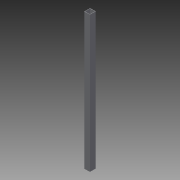
# Autodesk Inventor part: Edge Mount Interference
Saved by Autodesk Inventor 2013 (Build 170138000, 138)
## iProperties
Created: 2013-01-23
Part Number: Edge Mount Interference
Material: Generic
Document SubType Name: Modeling
Designer: actoennies
Density: 1 g/cm^3
Author: actoennies
Autodesk Inventor part; units mm, degrees
ref_plane "YZ Plane" through (0, 0, 0) normal (1, 0, 0) x (0, 1, 0)
ref_plane "XZ Plane" through (0, 0, 0) normal (0, 1, 0) x (-1, 0, 0)
ref_plane "XY Plane" through (0, 0, 0) normal (0, 0, 1) x (1, 0, 0)
sketch "Sketch1" plane through (0, 0, 0) normal (0, 1, 0) x (-1, 0, 0)
  line L0 (0, 0) -> (-25.4, 0)
  line L1 (-25.4, 0) -> (-25.4, 25.4)
  line L2 (-25.4, 25.4) -> (0, 25.4)
  line L3 (0, 25.4) -> (0, 0)
  line L4 (-1.5875, 23.8125) -> (-23.8125, 23.8125)
  line L5 (-23.8125, 23.8125) -> (-23.8125, 1.5875)
  line L6 (-23.8125, 1.5875) -> (-1.5875, 1.5875)
  line L7 (-1.5875, 1.5875) -> (-1.5875, 23.8125)
  dimension "d0" = 25.4
  dimension "d2" = 25.4
  dimension "d3" = 1.5875
  constraints: 16 end point, 4 parallel, 2 perpendicular, 1 horizontal, 3 other
  measures "d0" distance of L1.end L2.end
  measures "d2" distance of L2.end L0.start
  measures "d3" distance between parallel lines of L2 L4
extrude "Extrusion1" add sketch "Sketch1" along normal blind 914.4
sketch "Sketch2" plane through (0, 0, 25.4) normal (0, 0, 1) x (1, 0, 0)
  line L0 (25.4, 0) -> (0, 0) projected
  line L1 (25.4, 0) -> (25.4, 914.4) projected
  line L2 (0, 914.4) -> (25.4, 914.4) projected
  line L3 (0, 0) -> (0, 914.4) projected
  line L4 (0, 0) -> (25.4, 1.0809)
  line L5 (0, 597.4402) -> (25.4, 598.521)
  dimension "d6" = 596.9
  dimension "d7" = 597.4402
  constraints: 4 end point, 3 point on line, 1 parallel
  measures "d6" distance between parallel lines of L4 L5
  measures "d7" distance of L0.end L5.start
extrude "Extrusion2" cut sketch "Sketch2" against normal blind 914.4 contours L0 L4 L1 | L3 L2 L1 L5
body "Solid1"
